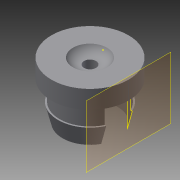
# Autodesk Inventor part: Cable end barrel stop
Saved by Autodesk Inventor 2014 SP2 (Build 180246200, 246)
## iProperties
Created: 2014-08-06
Part Number: Cable end barrel stop
Material: Generic
Document SubType Name: Modeling
Designer: Lukasz Szmit
Density: 1 g/cm^3
Appearance: Default
Author: Lukasz Szmit
Autodesk Inventor part; units mm, degrees
ref_plane "XZ Plane" through (0, 0, 0) normal (0, 1, 0) x (-1, 0, 0)
ref_plane "XY Plane" through (0, 0, 0) normal (0, 0, 1) x (1, 0, 0)
sketch "Sketch1" plane through (0, 0, 0) normal (0, 0, 1) x (1, 0, 0)
  circle A0 centre (0, 0) radius 6.4
  dimension "d0" = 12.8
  constraints: 1 centre point, 1 coincident
  measures "d0" diameter of A0
sketch "Sketch2" plane through (0, 0, 0) normal (0, 0, 1) x (1, 0, 0)
  circle A0 centre (0, 0) radius 2.825
  dimension "d3" = 5.65
  constraints: 1 centre point, 1 coincident
  measures "d3" diameter of A0
sketch "Sketch3" plane through (0, 0, 0) normal (0, 0, 1) x (1, 0, 0)
  circle A0 centre (0, 0) radius 1
  dimension "d4" = 2
  constraints: 1 centre point, 1 coincident
  measures "d4" diameter of A0
extrude "Extrusion1" add sketch "Sketch1" against normal blind 3
extrude "Extrusion2" cut sketch "Sketch2" against normal blind 1
extrude "Extrusion3" cut sketch "Sketch3" against normal blind 3
fillet "Fillet1" radius 2 1 edges at (-2.825, 0, -1)
sketch "Sketch4" plane through (0, 0, 0) normal (0, 1, 0) x (-1, 0, 0)
  line L0 (-5.0465, -3) -> (-5.0465, -6.35)
  line L1 (-6.4, -3) -> (6.4, -3) projected
  line L2 (-5.2965, -6.35) -> (-4.5465, -9.35)
  line L3 (-5.2965, -6.35) -> (-5.0465, -6.35)
  line L4 (-4.5465, -3) -> (-4.5465, -9.35)
  line L5 (-5.0465, -3) -> (-4.5465, -3)
  line L6 (0, -3) -> (0, -11.7949)
  point P0 (0, 0)
  dimension "d21" = 0.25
  dimension "d26" = 6.35
  dimension "d28" = 0.5
  dimension "d29" = 90
  constraints: 12 end point, 1 midpoint, 1 parallel, 1 perpendicular, 1 point on line
  measures "d21" distance from line of L0 L2.start
  measures "d26" distance of L4.start L2.end
  measures "d28" distance between parallel lines of L0 L4
  measures "d29" angle of L0 L3
revolve "Revolution2" add sketch "Sketch4" angle 360 about axis through (0, 0, -3) along (0, 0, -1)
ref_plane "Work Plane2" through (6.4, 0, 0) normal (1, 0, 0) x (0, 1, 0)
sketch "Sketch7" plane through (6.4, 0, 0) normal (1, 0, 0) x (0, 1, 0)
  line L0 (-2.15, -3) -> (-2.15, -9.35)
  line L1 (-2.15, -9.35) -> (2.15, -9.35)
  line L2 (2.15, -9.35) -> (2.15, -3)
  line L3 (2.15, -3) -> (-2.15, -3)
  point P0 (0, 0)
  dimension "d34" = 4.3
  dimension "d35" = 6.35
  constraints: 8 end point, 2 parallel, 1 perpendicular
  measures "d34" distance of L2.end L0.start
  measures "d35" distance of L0.start L0.end
extrude "Extrusion4" cut sketch "Sketch7" against normal blind 12.8
sketch "Sketch8" plane through (4.006, 2.15, -3) normal (0, -1, 0) x (1, 0, 0)
  line L0 (0, -6.35) -> (0, 0) projected
  line L1 (0.5596, -3.35) -> (0.8345, -3.35) projected
  line L2 (0.5596, 0) -> (0.5596, -3.35) projected
  line L3 (0.5596, 0) -> (0, 0) projected
  point P0 (-4.006, 3)
  constraints: 1 other
fillet "Fillet2" radius 1 2 edges at (0, 4.5465, -3) (0, -4.5465, -3)
fillet "Fillet3" radius 1 8 edges at (-3.4132, -2.15, -3) (-4.2858, -2.15, -3) (-3.4132, 2.15, -3) (-4.2858, 2.15, -3) (3.4132, 2.15, -3) (4.2858, 2.15, -3) (3.4132, -2.15, -3) (4.2858, -2.15, -3)
body "Solid1"
